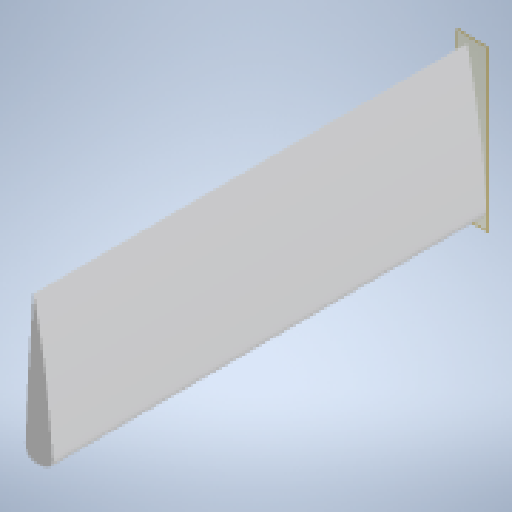
# Autodesk Inventor part: Vtail
Saved by Autodesk Inventor 2026 (Build 300175050, 175E)
## iProperties
Created: 2025-07-28
Part Number: Vtail
Material: Generic
Document SubType Name: Modeling
Designer: Cupri
Density: 1 g/cm^3
Appearance: Default
Author: Cupri
Autodesk Inventor part; units mm, degrees
ref_plane "YZ Plane" through (0, 0, 0) normal (1, 0, 0) x (0, 1, 0)
ref_plane "XZ Plane" through (0, 0, 0) normal (0, 1, 0) x (-1, 0, 0)
ref_plane "Work Plane1" through (0, 0, 0) normal (0, 0, 1) x (1, 0, 0)
sketch "Sketch1" plane through (0, 0, 0) normal (0, 0, 1) x (1, 0, 0)
  spline S0 degree 3 poles (-11.6918, 0.3474) (-9.6831, -8.2875) (-6.6853, -25.1621) (-2.182, -52.1537) (-0.1114, -65.8347) (3.0568, -94.1973) (4.2902, -107.6271) (5.2049, -120.5244) (5.4098, -123.4703) (5.6104, -127.2227) knots -42.934618 -42.934618 -42.934618 -42.934618 -30.454804 -30.454804 -15.874187 -15.874187 -5.406476 -5.406476 -3.702732 -3.702732 -3.702732 -3.702732 projected
  line L0 (-11.6918, 0.3474) -> (-12.268, 0.3645) projected
  spline S1 degree 3 poles (-19.7592, -126.469) (-19.1855, -111.8761) (-18.4212, -96.7836) (-15.3434, -44.9452) (-12.9313, -15.4603) (-12.268, 0.3645) knots -6.864026 -6.864026 -6.864026 -6.864026 -4.751617 -4.751617 0 0 0 0 projected
  line L1 (5.6104, -127.2227) -> (-19.7592, -126.469) projected
  point P0 (0, 0)
ref_plane "Work Plane2" through (-23.668, -128.0007, 381) normal (0, 0, -1) x (0, 1, 0)
extrude "Extrusion1" add sketch "Sketch1" along normal up to surface (381 mm away)
fillet "Fillet1" radius 9.525 2 edges at (5.6104, -127.2227, 190.5) (-19.7592, -126.469, 190.5)
body "Solid1"
